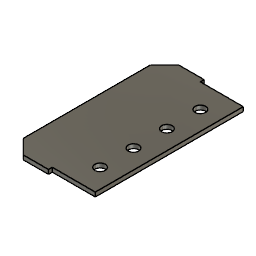
GPL H350 to 350G27_ (Autodesk Fusion 360 design; units mm, degrees)
Autodesk Fusion 360 part; units mm, degrees
sketch "スケッチ1" plane through (0, 0, 0) normal (0, 0, 1) x (1, 0, 0)
  line L0 (-3.5, 163) -> (-86.5, 163)
  line L1 (-86.5, 163) -> (-86.5, -163)
  line L2 (-86.5, -163) -> (-3.5, -163)
  line L3 (86.5, -155) -> (86.5, 155)
  line L4 (82.2546, 155) -> (-86.5, -163) construction
  line L5 (-86.5, 163) -> (82.2546, -155) construction
  line L6 (-3.5, 163) -> (-3.5, 155)
  line L7 (-3.5, 155) -> (86.5, 155)
  line L8 (-3.5, -163) -> (-3.5, -155)
  line L9 (-3.5, -155) -> (86.5, -155)
  dimension "d2" = 326
  constraint horizontal L0
  constraint perpendicular L0 L1
  constraint parallel L0 L2
  constraint parallel L1 L3
  constraint coincident L4 origin
  constraint coincident L5 origin
  constraint vertical L6
  constraint horizontal L7
  constraint vertical L8
  constraint horizontal L9
  constraint coincident L7 L4.start
  constraint coincident L9 L5.end
  measures "d2" distance of L0.end L1.end
extrude "押し出し1" add sketch "スケッチ1" along normal blind 9
chamfer "面取り1" distance 30 angle 45 2 edges at (-86.5, -163, 4.5) (-86.5, 163, 4.5)
sketch "スケッチ2" plane through (0, 0, 9) normal (0, 0, 1) x (-1, 0, 0)
  line L0 (56.5, -163) -> (86.5, -133)
  line L1 (86.5, -133) -> (86.5, 133)
  line L2 (86.5, 133) -> (56.5, 163)
  line L3 (56.5, 163) -> (3.5, 163)
  line L4 (3.5, 163) -> (3.5, 155)
  line L5 (3.5, 155) -> (-86.5, 155)
  line L6 (-86.5, 155) -> (-86.5, -155)
  line L7 (-86.5, -155) -> (3.5, -155)
  line L8 (3.5, -155) -> (3.5, -163)
  line L9 (3.5, -163) -> (56.5, -163)
  line L10 (-86.5, -155) -> (-46.5, -155) construction
  line L11 (-46.5, -155) -> (-46.5, -105) construction
  line L12 (-46.5, -105) -> (-86.5, -105) construction
  line L13 (-86.5, -105) -> (-86.5, -155) construction
  line L14 (-46.5, -105) -> (-46.5, -35) construction
  line L15 (-86.5, 0) -> (101.7247, 0)
  point P0 (-46.5, -105)
  point P1 (-46.5, -35)
  point P2 (-46.5, 105)
  point P3 (-46.5, 35)
  dimension "d10" = 40
  dimension "d11" = 50
  dimension "d12" = 70
  constraint horizontal L10
  constraint vertical L11
  constraint horizontal L12
  constraint vertical L13
  constraint coincident L6.end L7.start
  constraint perpendicular L12 L14
  constraint midpoint L6 L15.start
  constraint perpendicular L1 L15
  constraint coincident P0 L11.end
  constraint coincident P1 L14.end
  constraint symmetric P0 L15 P2
  constraint symmetric L15 P1 P3
  measures "d10" distance of L6.end L10.end
  measures "d11" distance of L6.end L12.end
  measures "d12" distance of P0 P1
hole "穴1" at (46.5, 105, 9) at (46.5, 35, 9) at (46.5, -35, 9) at (46.5, -105, 9) direction (0, 0, -1) diameter 22 end through all
